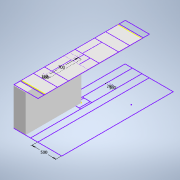
# Autodesk Inventor part: Marcoesumadre
Saved by Autodesk Inventor 2021.2 (Build 252289000, 289)
## iProperties
Created: 2021-04-11
Part Number: Marcoesumadre
Material: Genérico
Document SubType Name: Modeling
Designer: equip
Density: 1 g/cm^3
Appearance: Valor por defecto
Author: equip
Autodesk Inventor part; units mm, degrees
ref_plane "YZ Plane" through (0, 0, 0) normal (1, 0, 0) x (0, 1, 0)
ref_plane "XZ Plane" through (0, 0, 0) normal (0, 1, 0) x (-1, 0, 0)
ref_plane "XY Plane" through (0, 0, 0) normal (0, 0, 1) x (1, 0, 0)
sketch "Boceto1" plane through (0, 0, 0) normal (0, 1, 0) x (-1, 0, 0)
  line L0 (250.06, 997.344) -> (-249.94, 997.344)
  line L1 (-249.94, 997.344) -> (-249.94, -1002.656)
  line L2 (-249.94, -1002.656) -> (250.06, -1002.656)
  line L3 (250.06, -1002.656) -> (250.06, 997.344)
  point P0 (0, 0)
  point P1 (-115.972, 0)
  point P2 (-115.972, 0)
  point P3 (250.06, -1002.656)
  dimension "d0" = 2000
  dimension "d1" = 500
  constraints: 8 end point, 2 parallel, 1 coincident, 1 horizontal, 1 perpendicular
  measures "d0" distance of L3.start L0.start
  measures "d1" distance of L0.end L0.start
extrude "Extrusión1" add sketch "Boceto1" along normal blind 20
sketch "Boceto2" plane through (0, 20, 0) normal (0, 1, 0) x (1, 0, 0)
  line L0 (249.94, 1002.656) -> (-250.06, 1002.656) projected
  line L1 (-250.06, -749.844) -> (249.94, -749.844)
  line L2 (-250.06, -519.844) -> (249.94, -519.844)
  line L3 (-250.06, -114.844) -> (249.94, -114.844) construction
  line L4 (-250.06, 115.156) -> (249.94, 115.156)
  line L5 (-250.06, 520.156) -> (249.94, 520.156)
  line L6 (-250.06, 750.156) -> (249.94, 750.156)
  line L7 (-250.06, -997.344) -> (249.94, -997.344) projected
  line L8 (-250.06, -1154.844) -> (249.94, -1154.844)
  line L9 (-65.06, -62.344) -> (-65.06, 62.656)
  line L10 (64.94, 62.656) -> (64.94, -62.344)
  line L11 (249.94, -1024.844) -> (-250.06, -1024.844)
  line L12 (249.94, 1030.156) -> (-250.06, 1030.156)
  line L13 (249.94, 1160.156) -> (-250.06, 1160.156)
  line L14 (249.94, -1154.844) -> (249.94, 1160.156)
  line L15 (-250.06, -1154.844) -> (-250.06, 1160.156)
  line L16 (64.94, -62.344) -> (64.94, -114.844)
  line L17 (64.94, 62.656) -> (64.94, 115.156)
  line L18 (-65.06, 62.656) -> (-65.06, 115.156)
  line L19 (-65.06, -62.344) -> (-65.06, -114.844)
  line L20 (0, 0) -> (0, -700) construction
  line L21 (0, -647.8741) -> (-150, -647.8741) construction
  line L22 (-75, 2.656) -> (-250.06, 2.656) construction
  line L23 (0, -647.8741) -> (-100, -647.8741) construction
  line L24 (0, -647.8741) -> (100, -647.8741) construction
  line L25 (100, -519.844) -> (100, -114.844)
  line L26 (100, 115.156) -> (100, 520.156)
  dimension "d21" = 700
  dimension "d23" = 150
  dimension "d28" = 100
  dimension "d34" = 100
  constraints: 50 end point, 12 point on line, 4 perpendicular, 3 parallel, 2 horizontal, 2 vertical, 1 midpoint
  measures "d21" distance of L20.start L20.end
  measures "d23" distance of L21.start L21.end
  measures "d28" distance of L21.start L23.end
  measures "d34" distance of L21.start L24.end
sketch "Boceto3" plane through (0, 0, 0) normal (0, -1, 0) x (1, 0, 0)
  line L0 (0, 0) -> (-250.06, 0)
  line L1 (-250.06, 0) -> (-250.06, 1154.844)
  line L2 (-250.06, 1154.844) -> (0, 1154.844)
  line L3 (0, 1154.844) -> (0, 0)
  constraints: 8 end point, 2 parallel, 1 horizontal, 1 perpendicular
extrude "Extrusión2" add sketch "Boceto3" along normal blind 773
sketch "Boceto4" plane through (0, -773, 0) normal (0, -1, 0) x (1, 0, 0)
  line L0 (249.94, -1154.844) -> (249.94, 1160.156)
  line L1 (-250.06, -1154.844) -> (-250.06, 1160.156)
  line L2 (249.94, 1160.156) -> (-250.06, 1160.156)
  line L3 (-250.06, -1154.844) -> (249.94, -1154.844)
  line L4 (-65.06, -62.344) -> (-65.06, -114.844)
  line L5 (-65.06, 62.656) -> (-65.06, 115.156)
  line L6 (64.94, 62.656) -> (64.94, 115.156)
  line L7 (-65.06, -62.344) -> (-65.06, 62.656)
  line L8 (64.94, 62.656) -> (64.94, -62.344)
  line L9 (64.94, -62.344) -> (64.94, -114.844)
  line L10 (-100, -519.844) -> (-100, -1154.844) construction
  line L11 (-100, -1154.844) -> (-100, 1160.156)
  line L12 (100, -1154.844) -> (100, 1160.156)
  line L13 (249.94, 1160.156) -> (749.94, 1160.156)
  line L14 (749.94, 1160.156) -> (749.94, -1154.844)
  line L15 (749.94, -1154.844) -> (249.94, -1154.844)
  line L16 (0, -647.8741) -> (100, -647.8741) construction
  line L17 (100, -647.8741) -> (-100, -647.8741) construction
  line L18 (100, -647.8741) -> (100, -1154.844) construction
  line L19 (-100, -647.8741) -> (-100, -1154.844) construction
  line L20 (-100, 115.156) -> (100, 115.156)
  line L21 (-100, -114.844) -> (100, -114.844)
  point P0 (0, 0)
  point P1 (550.0765, -485.6293)
  dimension "d31" = 500
  dimension "d32" = 100
  dimension "d33" = 200
  constraints: 44 end point, 9 point on line, 7 perpendicular, 1 horizontal, 1 parallel, 1 vertical
  measures "d31" distance of L0.end L13.end
  measures "d32" distance of L16.start L16.end
  measures "d33" distance of L16.end L17.end
